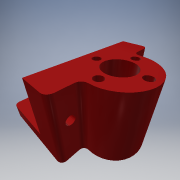
# Autodesk Inventor part: Z nut mount
Saved by Autodesk Inventor 2017 (Build 210142000, 142)
## iProperties
Part Number: Z nut mount
Material: ABS-Kunststoff
Document SubType Name: Modeling
Designer: Till
Density: 1.06 g/cm^3
Appearance: Rot
Author: Till
Autodesk Inventor part; units mm, degrees
ref_plane "YZ Plane" through (0, 0, 0) normal (1, 0, 0) x (0, 1, 0)
ref_plane "XZ Plane" through (0, 0, 0) normal (0, 1, 0) x (-1, 0, 0)
ref_plane "XY Plane" through (0, 0, 0) normal (0, 0, 1) x (1, 0, 0)
sketch "Skizze1" plane through (0, 0, 0) normal (0, 0, 1) x (1, 0, 0)
  line L0 (0, 20) -> (10, 20)
  line L1 (10, 20) -> (10, 10.735)
  arc A0 (10, -10.735) -> (10, 10.735) centre (12.4, 0) ccw
  line L2 (0, 20) -> (0, -20)
  line L3 (0, -20) -> (10, -20)
  line L4 (10, -20) -> (10, -10.735)
  circle A1 centre (12.4, 0) radius 5.2
  point P0 (0, 0)
  dimension "d0" = 10
  dimension "d1" = 40
  dimension "d2" = 10
  dimension "d3" = 11
  dimension "d4" = 0
  dimension "d5" = 20
  dimension "d6" = 10.4
  dimension "d7" = 12.4
  constraints: 10 end point, 3 perpendicular, 2 centre point, 2 point on circle, 1 coincident, 1 horizontal, 1 vertical
  measures "d0" distance of L0.start L0.end
  measures "d1" distance of L0.start L2.end
  measures "d2" distance of L2.end L3.end
  measures "d3" radius of A0
  measures "d4" vertical distance of point (0, 0) A0.centre
  measures "d5" distance from line of point (0, 0) L0
  measures "d6" diameter of A1
  measures "d7" distance from line of L2 A0.centre
extrude "Extrusion1" add sketch "Skizze1" along normal blind 25
sketch "Skizze2" plane through (0, -20, 0) normal (-1, 0, 0) x (0, 0, 1)
  line L0 (0, 0) -> (25, 0) projected
  line L1 (0, 40) -> (5, 40)
  line L2 (5, 40) -> (5, 0)
  line L3 (5, 0) -> (0, 0)
  line L4 (0, 0) -> (0, 40)
  point P0 (0, 20)
  dimension "d10" = 5
  constraints: 8 end point, 2 parallel, 1 horizontal, 1 perpendicular, 1 point on line
  measures "d10" distance of L2.end L3.end
extrude "Extrusion2" add sketch "Skizze2" along normal blind 20
sketch "Skizze3" plane through (0, 0, 0) normal (0, 0, -1) x (-1, 0, 0)
  circle A0 centre (10, -10) radius 1.6
  circle A1 centre (10, 10) radius 1.6
  line L0 (-10, -20) -> (20, -20) projected
  line L1 (20, 20) -> (20, -20) projected
  line L2 (20, 20) -> (-10, 20) projected
  point P0 (0, 0)
  dimension "d13" = 3.2
  dimension "d14" = 3.2
  dimension "d15" = 10
  dimension "d16" = 10
  dimension "d17" = 10
  dimension "d18" = 10
  constraints: 2 centre point
  measures "d13" diameter of A0
  measures "d14" diameter of A1
  measures "d15" distance from line of L0 A0.centre
  measures "d16" distance from line of L1 A0.centre
  measures "d17" distance from line of L2 A1.centre
  measures "d18" distance from line of L1 A1.centre
extrude "Extrusion3" cut sketch "Skizze3" against normal through all
fillet "Rundung1" radius 2 6 edges at (10, 20, 12.5) (10, 10.735, 12.5) (10, -10.735, 12.5) (10, -20, 12.5) (-20, -20, 2.5) (-20, 20, 2.5)
sketch "Skizze4" plane through (10, -18, 0) normal (1, 0, 0) x (0, 0, -1)
  circle A0 centre (-15, 3) radius 1.6
  circle A1 centre (-15, 33) radius 1.6
  line L0 (-25, -2) -> (0, -2) projected
  line L1 (-25, 0) -> (-25, 5.0062) projected
  line L2 (0, 38) -> (-25, 38) projected
  line L3 (-25, 30.9938) -> (-25, 36) projected
  point P0 (0, 18)
  dimension "d22" = 3.2
  dimension "d23" = 3.2
  dimension "d24" = 5
  dimension "d25" = 10
  dimension "d26" = 5
  dimension "d27" = 10
  constraints: 2 centre point
  measures "d22" diameter of A0
  measures "d23" diameter of A1
  measures "d24" distance from line of L0 A0.centre
  measures "d25" distance from line of L1 A0.centre
  measures "d26" distance from line of L2 A1.centre
  measures "d27" distance from line of L3 A1.centre
extrude "Extrusion4" cut sketch "Skizze4" against normal through all
sketch "Skizze5" plane through (0, 0, 25) normal (0, 0, 1) x (1, 0, 0)
  circle A0 centre (4.4, 0) radius 1.5
  circle A1 centre (12.4, 0) radius 5.2 construction
  circle A2 centre (12.4, -8) radius 1.5
  circle A3 centre (20.4, 0) radius 1.5
  circle A4 centre (12.4, 8) radius 1.5
  point P0 (0, 0)
  dimension "d30" = 3
  dimension "d31" = 8
  dimension "d34" = 360
  constraints: 4 centre point, 9 other
  measures "d30" diameter of A0
  measures "d31" distance of A1.centre A0.centre
extrude "Extrusion5" cut sketch "Skizze5" against normal blind 20
